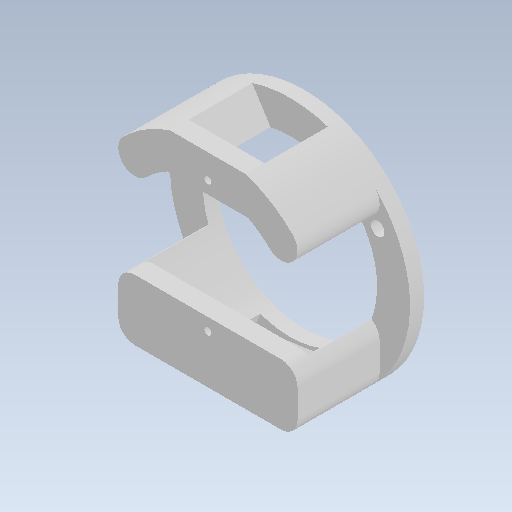
# Autodesk Inventor part: Soporte_Servo
Saved by Autodesk Inventor 2020.1 (Build 241239000, 239)
## iProperties
Created: 2019-12-05
Part Number: Soporte_Servo
Material: Generic
Document SubType Name: Modeling
Designer: Daniel
Density: 1 g/cm^3
Appearance: Default
Author: Daniel
Autodesk Inventor part; units mm, degrees
ref_plane "YZ Plane" through (0, 0, 0) normal (1, 0, 0) x (0, 1, 0)
ref_plane "XZ Plane" through (0, 0, 0) normal (0, 1, 0) x (-1, 0, 0)
ref_plane "XY Plane" through (0, 0, 0) normal (0, 0, 1) x (1, 0, 0)
sketch "Sketch1" plane through (0, 0, 0) normal (0, 0, 1) x (1, 0, 0)
  circle A0 centre (-21.5, 0) radius 1.25
  circle A1 centre (21.5, 0) radius 1.25
  circle A2 centre (0, 21.5) radius 1.25
  circle A3 centre (0, -21.5) radius 1.25
  circle A4 centre (0, 0) radius 25.5
  circle A5 centre (0, 0) radius 17.5
  circle A6 centre (0, 0) radius 18.5
  circle A7 centre (0, -21.5) radius 1.45
  circle A8 centre (18.619546, 10.75) radius 1.45
  circle A9 centre (-18.619546, 10.75) radius 1.45
  dimension "d0" = 1
  dimension "d28" = 0.2
  dimension "d31" = 360
  constraints: 4 centre point, 2 coincident, 7 other
  measures "d0" radial gap between concentric circles of A5 A6
  measures "d28" radial gap between concentric circles of A7 A3
extrude "Extrusion1" add sketch "Sketch1" along normal blind 3 contours A0 | A1 | A2 | A4
sketch "Sketch2" plane through (0, 0, 3) normal (0, 0, 1) x (1, 0, 0)
  circle A0 centre (0, 21.5) radius 1.45 construction
  line L0 (0, 0) -> (15.556349, 15.556349) construction
  line L1 (0, 0) -> (38.538256, 0) construction
  circle A1 centre (0, 0) radius 25.5
  line L2 (-25.5, 0) -> (-18.5, 0) construction
  circle A2 centre (0, 0) radius 18.5
  circle A3 centre (0, 0) radius 22 construction
  circle A4 centre (15.556349, 15.556349) radius 3.5
  circle A5 centre (-15.556349, 15.556349) radius 3.5
  circle A6 centre (-15.556349, -15.556349) radius 3.5
  circle A7 centre (15.556349, -15.556349) radius 3.5
  dimension "d9" = 44
  dimension "d8" = 45
  dimension "d12" = 360
  constraints: 6 end point, 4 centre point, 3 coincident, 2 horizontal, 2 horizontal alignment, 14 other
  measures "d8" angle of L1 L0
extrude "Extrusion2" add sketch "Sketch2" along normal blind 17.45 contours A4 | A7 | A5 | A6
sketch "Sketch3" plane through (15.556349, 15.556349, 20.45) normal (0, 0, 1) x (1, 0, 0)
  line L0 (-10.306349, -21.656349) -> (-20.806349, -21.656349)
  line L1 (-20.806349, 0.843651) -> (-10.306349, 0.843651)
  arc A0 (-28.637825, -2.474874) -> (-33.587572, 2.474874) centre (-31.112698, 0) ccw
  line L2 (-27.715898, 0.843651) -> (-3.3968, 0.843651)
  line L3 (3.5, -21.656349) -> (-34.612698, -21.656349)
  line L4 (3.5, -21.656349) -> (3.5, -31.112698)
  line L5 (0, -34.612698) -> (-31.112698, -34.612698)
  line L6 (-34.612698, -31.112698) -> (-34.612698, -21.656349)
  circle A1 centre (0, -31.112698) radius 3.5
  circle A2 centre (-31.112698, -31.112698) radius 3.5
  circle A3 centre (0, -31.112698) radius 3.5
  circle A4 centre (-31.112698, -31.112698) radius 3.5
  line L7 (3.5, 0) -> (3.5, 8.643651)
  line L8 (3.5, 8.643651) -> (-34.612698, 8.643651)
  line L9 (-34.612698, 8.643651) -> (-34.612698, 0)
  circle A5 centre (-31.112698, 0) radius 3.5
  circle A6 centre (0, 0) radius 3.5
  line L10 (-20.806349, 5.643651) -> (-16.106349, 5.643651)
  point P0 (-15.556349, -15.556349)
  point P1 (0, -34.612698)
  point P2 (-10.306349, 0.843651)
  dimension "d16" = 3
  constraints: 16 end point, 8 point on circle, 5 tangent, 4 perpendicular, 2 collinear, 2 horizontal, 2 vertical
  measures "d16" distance between parallel lines of L8 L10
extrude "Extrusion3" add sketch "Sketch3" against normal blind 4
fillet "Fillet1" radius 3.5 4 edges at (19.0563, 24.2, 18.45) (19.0563, -6.1, 18.45) (-19.0563, -6.1, 18.45) (-19.0563, 24.2, 18.45)
sketch "Sketch4" plane through (15.556349, 15.556349, 16.45) normal (0, 0, -1) x (-1, 0, 0)
  circle A0 centre (15.556349, 3.493651) radius 2.4
  circle A1 centre (15.556349, -24.306349) radius 2.4
  point P0 (15.556349, -15.556349)
  constraints: 2 coincident
hole "Hole1" at (0, -8.75, 16.45) at (0, 19.05, 16.45) direction (0, 0, 1) diameter 1.5 depth 10 tip angle 118
sketch "Sketch5" plane through (0, 0, 3) normal (0, 0, 1) x (1, 0, 0)
  arc A0 (18.031223, 18.031223) -> (13.081475, 13.081475) centre (15.556349, 15.556349) ccw
  arc A1 (18.031223, 18.031223) -> (-18.031223, 18.031223) centre (0, 0) ccw
  arc A2 (-13.081475, 13.081475) -> (-18.031223, 18.031223) centre (-15.556349, 15.556349) ccw
  arc A3 (13.081475, 13.081475) -> (-13.081475, 13.081475) centre (0, 0) ccw
  circle A4 centre (0, 19.05) radius 0.75
  arc A5 (-15.556349, 24.2) -> (-19.056349, 20.7) centre (-15.556349, 20.7) ccw
  line L0 (-19.056349, 20.7) -> (-19.056349, 15.556349)
  arc A6 (-19.056349, 15.556349) -> (-12.159549, 16.4) centre (-15.556349, 15.556349) ccw
  line L1 (-12.159549, 16.4) -> (12.159549, 16.4)
  arc A7 (12.159549, 16.4) -> (19.056349, 15.556349) centre (15.556349, 15.556349) ccw
  line L2 (19.056349, 15.556349) -> (19.056349, 20.7)
  arc A8 (19.056349, 20.7) -> (15.556349, 24.2) centre (15.556349, 20.7) ccw
  line L3 (15.556349, 24.2) -> (-15.556349, 24.2)
  arc A9 (18.031223, 18.031223) -> (-18.031223, 18.031223) centre (0, 0) ccw
  line L4 (8.038035, 24.2) -> (4.138236, 18.031223)
  arc A10 (13.081475, 13.081475) -> (-13.081475, 13.081475) centre (0, 0) ccw
  line L5 (-8.038035, 24.2) -> (-4.138236, 18.031223)
  point P0 (8.038035, 24.2)
  point P1 (-8.038035, 24.2)
  point P2 (-0.502441, 18.493176)
  point P3 (0.502441, 18.493176)
  point P4 (-12.159549, 16.4)
  point P5 (-8.560958, 16.4)
  point P6 (8.038035, 24.2)
  constraints: 4 end point, 4 point on circle, 2 point on line
extrude "Extrusion4" add sketch "Sketch5" along normal up to surface (17.45 mm away) contours A0 L1 A3 L4 A1 | A0 A3 L1 | L5 A3 L1 A2 A1 | A3 A2 L1
sketch "Sketch6" plane through (15.556349, 15.556349, 16.45) normal (0, 0, -1) x (-1, 0, 0)
  arc A0 (7.518315, 8.643651) -> (-2.474874, 2.474874) centre (15.556349, -15.556349) ccw
  line L0 (7.518315, 8.643651) -> (0, 8.643651)
  arc A1 (0, 8.643651) -> (-3.5, 5.143651) centre (0, 5.143651) ccw
  line L1 (-3.5, 5.143651) -> (-3.5, 0)
  arc A2 (-2.474874, 2.474874) -> (-3.5, 0) centre (0, 0) ccw
  arc A3 (33.587572, 2.474874) -> (23.594384, 8.643651) centre (15.556349, -15.556349) ccw
  arc A4 (34.612698, 0) -> (33.587572, 2.474874) centre (31.112698, 0) ccw
  line L2 (34.612698, 0) -> (34.612698, 5.143651)
  arc A5 (34.612698, 5.143651) -> (31.112698, 8.643651) centre (31.112698, 5.143651) ccw
  line L3 (31.112698, 8.643651) -> (23.594384, 8.643651)
extrude "Extrusion5" cut sketch "Sketch6" against normal blind 10
sketch "Sketch7" plane through (0, 0, 3) normal (0, 0, 1) x (1, 0, 0)
  circle A0 centre (0, -21.5) radius 1.45
  arc A1 (13.081475, -13.081475) -> (18.031223, -18.031223) centre (15.556349, -15.556349) ccw
  arc A2 (-13.081475, -13.081475) -> (13.081475, -13.081475) centre (0, 0) ccw
  arc A3 (-18.031223, -18.031223) -> (-13.081475, -13.081475) centre (-15.556349, -15.556349) ccw
  arc A4 (-18.031223, -18.031223) -> (18.031223, -18.031223) centre (0, 0) ccw
  arc A5 (18.031223, -18.031223) -> (13.081475, -13.081475) centre (15.556349, -15.556349) ccw
  arc A6 (18.031223, -18.031223) -> (18.031223, 18.031223) centre (0, 0) ccw
  arc A7 (13.081475, 13.081475) -> (18.031223, 18.031223) centre (15.556349, 15.556349) ccw
  arc A8 (13.081475, -13.081475) -> (13.081475, 13.081475) centre (0, 0) ccw
  circle A9 centre (18.619546, 10.75) radius 1.45
  arc A10 (-13.081475, -13.081475) -> (-18.031223, -18.031223) centre (-15.556349, -15.556349) ccw
  arc A11 (-13.081475, 13.081475) -> (-13.081475, -13.081475) centre (0, 0) ccw
  arc A12 (-18.031223, 18.031223) -> (-13.081475, 13.081475) centre (-15.556349, 15.556349) ccw
  arc A13 (-18.031223, 18.031223) -> (-18.031223, -18.031223) centre (0, 0) ccw
  circle A14 centre (-18.619546, 10.75) radius 1.45
  circle A15 centre (0, -8.75) radius 0.75
  arc A16 (-15.556349, -6.1) -> (-19.056349, -9.6) centre (-15.556349, -9.6) ccw
  line L0 (-19.056349, -9.6) -> (-19.056349, -15.556349)
  arc A17 (-19.056349, -15.556349) -> (-15.556349, -19.056349) centre (-15.556349, -15.556349) ccw
  line L1 (-15.556349, -19.056349) -> (15.556349, -19.056349)
  arc A18 (15.556349, -19.056349) -> (19.056349, -15.556349) centre (15.556349, -15.556349) ccw
  line L2 (19.056349, -15.556349) -> (19.056349, -9.6)
  arc A19 (19.056349, -9.6) -> (15.556349, -6.1) centre (15.556349, -9.6) ccw
  line L3 (15.556349, -6.1) -> (-15.556349, -6.1)
  arc A20 (-13.081475, -13.081475) -> (13.081475, -13.081475) centre (0, 0) ccw
  line L4 (-6.327373, -17.384313) -> (-8.721514, -23.962162)
  arc A21 (-18.031223, -18.031223) -> (18.031223, -18.031223) centre (0, 0) ccw
  line L5 (6.327373, -17.384313) -> (8.721514, -23.962162)
  line L6 (0, -21.5) -> (0, -25.5) construction
  point P0 (6.935944, -19.056349)
  point P1 (15.556349, -19.056349)
  point P2 (17.296616, -6.563312)
  point P3 (-6.935944, -19.056349)
  point P4 (-13.081475, -13.081475)
  point P5 (-13.081475, -13.081475)
  point P6 (-13.081475, -13.081475)
  point P7 (-13.081475, -13.081475)
  point P8 (-17.296616, -6.563312)
  dimension "d37" = 40
  dimension "d38" = 20
  constraints: 6 end point, 5 point on circle, 2 line through centre
  measures "d37" angle of L4 L5
  measures "d38" angle of L6 L5
extrude "Extrusion6" add sketch "Sketch7" along normal up to surface (17.45 mm away) contours A1 L1 L5 A2 | A8 A19 L2 A5 | L4 L1 A3 A2 | A10 L0 A16 A11
ref_plane "Work Plane1" through (15.556349, -19.056349, 3) normal (-0.7465912, -0.665283, 0) x (0, 0, 1)
sketch "Sketch8" plane through (15.556349, -19.056349, 3) normal (-0.7465912, -0.665283, 0) x (0, 0, 1)
  line L0 (13.45, 6.10728) -> (13.45, 17.354006)
  line L1 (13.45, 17.354006) -> (17.45, 17.354006)
  line L2 (17.45, 17.354006) -> (17.45, 0)
  line L3 (17.45, 0) -> (0, 0)
  line L4 (0, 0) -> (0, -0.901129)
  line L5 (0, -0.901129) -> (-3, -0.901129)
  line L6 (-3, -0.901129) -> (-3, 6.10728)
  line L7 (-3, 6.10728) -> (13.45, 6.10728)
  line L8 (17.45, 50.054486) -> (17.45, 43.046077)
  line L9 (17.45, 43.046077) -> (0, 43.046077)
  line L10 (0, 43.046077) -> (-3, 43.046077)
  line L11 (-3, 43.046077) -> (-3, 50.054486)
  line L12 (-3, 50.054486) -> (17.45, 50.054486)
  line L13 (13.45, 14.55728) -> (5, 6.10728)
  point P0 (-3, 24.576679)
  dimension "d41" = 8
  dimension "d49" = 45
  constraints: 2 end point, 2 point on line
  measures "d41" distance of L13.end L6.end
  measures "d49" angle of L7 L13
extrude "Extrusion7" add sketch "Sketch8" along normal blind 1 and the other way blind 2 contours L7 L13 L0
mirror "Mirror1" about plane through (0, 0, 0) normal (1, 0, 0) of "Extrusion7"
body "Solid1"
